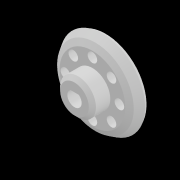
# Autodesk Inventor part: ShoulderMiterGear
Saved by Autodesk Inventor 2020 (Build 240168000, 168)
## iProperties
Created: 2021-01-27
Part Number: ShoulderMiterGear
Material: Generic
Document SubType Name: Modeling
Designer: valer
Density: 1 g/cm^3
Appearance: Default
Author: valer
Autodesk Inventor part; units mm, degrees
ref_plane "YZ Plane" through (0, 0, 0) normal (1, 0, 0) x (0, 1, 0)
ref_plane "XZ Plane" through (0, 0, 0) normal (0, 1, 0) x (-1, 0, 0)
sketch "Sketch1" plane through (0, 0, 0) normal (0, 0, 1) x (1, 0, 0)
  circle A0 centre (0, 0) radius 18.65
  dimension "d0" = 37.3
  constraints: 1 centre point, 1 coincident
  measures "d0" diameter of A0
ref_plane "Work Plane1" through (0, 0, 5.5) normal (0, 0, 1) x (1, 0, 0)
sketch "Sketch2" plane through (0, 0, 5.5) normal (0, 0, 1) x (1, 0, 0)
  circle A0 centre (0, 0) radius 15.25
  dimension "d2" = 30.5
  constraints: 1 centre point, 1 coincident
  measures "d2" diameter of A0
loft "Loft1" add profiles "Sketch1", "Sketch2"
sketch "Sketch3" plane through (0, 0, 5.5) normal (0, 0, 1) x (1, 0, 0)
  circle A0 centre (0, 0) radius 3
  line L0 (0, 0) -> (0, -3) construction
  line L1 (-1.8, 2.4) -> (1.8, 2.4)
  dimension "d7" = 6
  dimension "d8" = 5.4
  constraints: 4 end point, 3 point on circle, 1 centre point, 1 coincident, 1 horizontal, 1 vertical
  measures "d7" diameter of A0
  measures "d8" distance from line of L0.end L1
extrude "Extrusion1" cut sketch "Sketch3" against normal through all contours A0 L1 picked at (0.3021, 0.4498)
chamfer "Chamfer1" distance 1.5 angle 45 1 edges at (-18.65, 0, 0)
chamfer "Chamfer2" distance 1.5 angle 45 1 edges at (-15.25, 0, 5.5)
sketch "Sketch4" plane through (0, 0, 5.5) normal (0, 0, 1) x (1, 0, 0)
  circle A0 centre (0, 0) radius 7.5
  arc A1 (-1.8, 2.4) -> (1.8, 2.4) centre (0, 0) ccw projected
  line L0 (-1.8, 2.4) -> (1.8, 2.4) projected
  dimension "d17" = 15
  constraints: 1 centre point, 1 coincident
  measures "d17" diameter of A0
extrude "Extrusion2" add sketch "Sketch4" along normal blind 7.5
chamfer "Chamfer3" distance 1.5 angle 45 1 edges at (-7.5, 0, 13)
sketch "Sketch5" plane through (0, 0, 5.5) normal (0, 0, 1) x (1, 0, 0)
  circle A0 centre (0, 11.3137) radius 2
  circle A1 centre (-8, 8) radius 2
  circle A2 centre (-8, -8) radius 2
  line L0 (-8, 8) -> (-8, -8) construction
  circle A3 centre (0, 0) radius 17.8613 projected
  line L1 (-17.8613, 0) -> (0, 0) construction
  circle A4 centre (-11.3137, 0) radius 2
  circle A5 centre (0, 0) radius 11.3137 construction
  line L2 (0, 0) -> (0, 17.8613) construction
  circle A6 centre (0, -11.3137) radius 2
  circle A7 centre (0, 0) radius 7.5 projected
  line L3 (0, 0) -> (0, -17.8613) construction
  circle A8 centre (8, 8) radius 2
  circle A9 centre (8, -8) radius 2
  circle A10 centre (11.3137, 0) radius 2
  point P0 (-8, 0)
  dimension "d23" = 4
  dimension "d24" = 16
  dimension "d25" = 16
  constraints: 9 centre point, 8 end point, 7 point on circle, 4 equal radius, 4 point on line, 3 symmetric about line, 3 vertical, 1 coincident, 1 horizontal, 1 midpoint, 3 other
  measures "d23" diameter of A0
  measures "d24" distance of L0.start L0.end
  measures "d25" distance of A9.centre L0.end
extrude "Extrusion3" cut sketch "Sketch5" against normal through all contours A0 | A1 | A2 | A4 | A6 | A8 | A9 | A10
body "Solid1"
